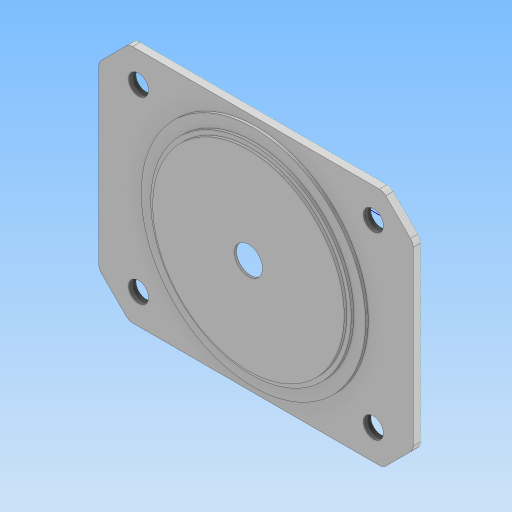
# Autodesk Inventor part: oberer_Rotierkörper_Rolle
Saved by Autodesk Inventor 2024.4 (Build 284460000, 460)
## iProperties
Created: 2026-01-07
Part Number: oberer_Rotierkörper_Rolle
Material: Generisch
Document SubType Name: Modeling
Designer: windows-desktop
Mass: 15.7018 g
Surface Area: 184.406 cm^2
Volume: 15.7018 cm^3
Density: 1 g/cm^3
Appearance: Vorgabe
Masse[kg]: 0,016 kg
Author: windows-desktop
Autodesk Inventor part; units mm, degrees
ref_plane "YZ Plane" through (0, 0, 0) normal (1, 0, 0) x (0, 1, 0)
ref_plane "XZ Plane" through (0, 0, 0) normal (0, 1, 0) x (-1, 0, 0)
ref_plane "XY Plane" through (0, 0, 0) normal (0, 0, 1) x (1, 0, 0)
sketch "Skizze1" plane through (0, 0, 0) normal (0, 1, 0) x (-1, 0, 0)
  line L0 (52.5, 40) -> (-52.5, 40)
  line L1 (-52.5, 40) -> (-52.5, -40)
  line L2 (-52.5, -40) -> (52.5, -40)
  line L3 (52.5, -40) -> (52.5, 40)
  line L4 (0, -56) -> (0, 56) construction
  line L5 (73.5, 0) -> (-73.5, 0) construction
  point P0 (0, 0)
  point P1 (-39.25, -30)
  point P2 (-39.25, 30)
  point P3 (39.25, -30)
  point P4 (39.25, 30)
  dimension "d0" = 105
  dimension "d1" = 80
  dimension "d2" = 39.25
  dimension "d3" = 30
  constraints: 8 end point, 3 symmetric about line, 2 parallel, 1 horizontal, 1 perpendicular, 2 other
  measures "d0" distance of L2.end L1.end
  measures "d1" distance of L1.end L0.end
  measures "d2" distance from line of L4 point (-39.25, -30)
  measures "d3" distance from line of L5 point (-39.25, -30)
extrude "Extrusion1" add sketch "Skizze1" against normal blind 2.5
hole "Bohrung1" at (39.25, 0, -30) at (39.25, 0, 30) at (-39.25, 0, 30) at (-39.25, 0, -30) direction (0, -1, 0) diameter 6.647 depth 14 tip angle 118 thread size "M8x1.25" class "6H" standard "ISO Metric profile"
chamfer "Fasen1" distance 10 angle 45 4 edges at (52.5, -1.25, 40) (52.5, -1.25, -40) (-52.5, -1.25, -40) (-52.5, -1.25, 40)
fillet "Rundung1" radius 3 8 edges at (-42.5, -1.25, 40) (-52.5, -1.25, 30) (-52.5, -1.25, -30) (-42.5, -1.25, -40) (42.5, -1.25, -40) (52.5, -1.25, -30) (42.5, -1.25, 40) (52.5, -1.25, 30)
sketch "Skizze2" plane through (0, -2.5, 0) normal (0, -1, 0) x (1, 0, 0)
  circle A0 centre (0, 0) radius 37.5
  circle A1 centre (0, 0) radius 34
  circle A2 centre (0, 0) radius 33.5
  circle A3 centre (0, 0) radius 32
  circle A4 centre (0, 0) radius 25
  circle A5 centre (0, 0) radius 23.5
  circle A6 centre (0, 0) radius 7.5
  circle A7 centre (0, 0) radius 6.5
  circle A8 centre (0, 0) radius 6
  circle A9 centre (0, 0) radius 4.5
  dimension "d17" = 75
  dimension "d18" = 68
  dimension "d19" = 67
  dimension "d20" = 64
  dimension "d21" = 50
  dimension "d22" = 47
  dimension "d23" = 15
  dimension "d24" = 13
  dimension "d25" = 12
  dimension "d26" = 9
  constraints: 10 centre point, 10 coincident
  measures "d17" diameter of A0
  measures "d18" diameter of A1
  measures "d19" diameter of A2
  measures "d20" diameter of A3
  measures "d21" diameter of A4
  measures "d22" diameter of A5
  measures "d23" diameter of A6
  measures "d24" diameter of A7
  measures "d25" diameter of A8
  measures "d26" diameter of A9
extrude "Extrusion2" cut sketch "Skizze2" against normal blind 2.5 contours A0 | A1 | A2 | A3 | A4 | A5 | A6 | A7 | A8 | A9
extrude "Extrusion3" add sketch "Skizze2" along normal blind 0.8333 contours A0 | A1
extrude "Extrusion5" add sketch "Skizze2" along normal blind 1.6666 contours A2
extrude "Extrusion6" add sketch "Skizze2" along normal blind 2.5 contours A3 | A4
sketch "Skizze3" plane through (0, -5, 0) normal (0, -1, 0) x (1, 0, 0)
  circle A0 centre (0, 0) radius 23.5 construction
  circle A1 centre (0, 0) radius 4.5
  circle A2 centre (0, 0) radius 6
  circle A3 centre (0, 0) radius 6.5
  circle A4 centre (0, 0) radius 7.5
  circle A5 centre (0, 0) radius 23.5
  circle A6 centre (0, 0) radius 32 construction
  circle A7 centre (0, 0) radius 4.65
  dimension "d37" = 9
  dimension "d38" = 12
  dimension "d39" = 13
  dimension "d40" = 15
  dimension "d47" = 9.3
  constraints: 6 centre point, 6 coincident
  measures "d37" diameter of A1
  measures "d38" diameter of A2
  measures "d39" diameter of A3
  measures "d40" diameter of A4
  measures "d47" diameter of A7
extrude "Extrusion7" add sketch "Skizze3" against normal blind 1 contours A5
extrude "Extrusion8" add sketch "Skizze3" against normal blind 0.75 contours A4
extrude "Extrusion9" add sketch "Skizze3" against normal blind 0.7 contours A3
extrude "Extrusion10" add sketch "Skizze3" against normal blind 0.65 contours A2
sketch "Skizze4" plane through (-52.5, 0, -28.7574) normal (-1, 0, 0) x (0, 0, 1)
  line L0 (0, -2.5) -> (0, 0) construction
  line L1 (57.5147, -2.5) -> (0, -2.5) construction
  line L2 (57.5147, 0) -> (57.5147, -2.5) construction
  line L3 (0, 0) -> (57.5147, 0) construction
  line L4 (-3.2426, -5) -> (60.7574, -5) construction
  point P0 (28.7574, 0)
  dimension "d53" = 2.5
  dimension "d54" = 5
  measures "d53" distance between parallel lines of L3 L1
  measures "d54" distance between parallel lines of L4 L3
sketch "Skizze5" plane through (0, 0, 0) normal (0, 1, 0) x (1, 0, 0)
  circle A0 centre (0, 0) radius 37.5 construction
  arc A1 (51.6213, -30.8787) -> (52.5, -28.7574) centre (49.5, -28.7574) ccw construction
  line L0 (52.5, -28.7574) -> (52.5, 28.7574) construction
  arc A2 (52.5, 28.7574) -> (51.6213, 30.8787) centre (49.5, 28.7574) ccw construction
  line L1 (43.3787, 39.1213) -> (51.6213, 30.8787) construction
  arc A3 (43.3787, 39.1213) -> (41.2574, 40) centre (41.2574, 37) ccw construction
  line L2 (41.2574, 40) -> (-41.2574, 40) construction
  arc A4 (-41.2574, 40) -> (-43.3787, 39.1213) centre (-41.2574, 37) ccw construction
  line L3 (-51.6213, 30.8787) -> (-43.3787, 39.1213) construction
  arc A5 (-51.6213, 30.8787) -> (-52.5, 28.7574) centre (-49.5, 28.7574) ccw construction
  line L4 (-52.5, 28.7574) -> (-52.5, -28.7574) construction
  arc A6 (-52.5, -28.7574) -> (-51.6213, -30.8787) centre (-49.5, -28.7574) ccw construction
  line L5 (-43.3787, -39.1213) -> (-51.6213, -30.8787) construction
  arc A7 (-43.3787, -39.1213) -> (-41.2574, -40) centre (-41.2574, -37) ccw construction
  line L6 (-41.2574, -40) -> (41.2574, -40) construction
  arc A8 (41.2574, -40) -> (43.3787, -39.1213) centre (41.2574, -37) ccw construction
  line L7 (51.6213, -30.8787) -> (43.3787, -39.1213) construction
  circle A9 centre (39.25, 30) radius 3.3235 construction
  circle A10 centre (39.25, -30) radius 3.3235 construction
  circle A11 centre (-39.25, -30) radius 3.3235 construction
  circle A12 centre (-39.25, 30) radius 3.3235 construction
  line L8 (39.25, -30) -> (0, -30)
  line L9 (0, -30) -> (0, 0)
  constraints: 4 end point, 1 horizontal, 1 perpendicular
